test modle freq v2 (Autodesk Fusion 360 design; units mm, degrees)
Autodesk Fusion 360 part; units mm, degrees
ref_plane "WorkPlane1" through (0, 28.011, 0) normal (0, 1, 0) x (0, 0, 1)
sketch "Sketch2" plane through (0, 28.011, 0) normal (0, 1, 0) x (1, 0, 0)
  line L0 (-47.6227, 0.6459) -> (-8.7892, -42.213)
  line L1 (-8.7892, -39.7251) -> (-48.648, 4.2654)
  line L2 (-8.7892, -42.213) -> (0, -42.213)
  line L3 (0, -42.213) -> (0, -36.199)
  line L4 (0, -36.199) -> (-8.7892, -36.199)
  line L5 (-8.7892, -36.199) -> (-8.7892, -42.213)
  line L6 (-47.6227, 0.6459) -> (0, 0.6459)
  line L7 (0, 0.6459) -> (0, 9.3893)
  line L8 (0, 9.3893) -> (-47.6227, 9.3893)
  line L9 (-47.6227, 9.3893) -> (-47.6227, 0.6459)
  constraint parallel L0 L1
  constraint horizontal L2
  constraint vertical L3
  constraint horizontal L4
  constraint vertical L5
  constraint horizontal L6
  constraint vertical L7
  constraint horizontal L8
  constraint vertical L9
  constraint coincident L5 L1.start
extrude "Extrude1" add sketch "Sketch2" along normal blind 3
extrude "Extrude2" add sketch "Sketch2" against normal up to surface (28.011 mm away) contours L1 L6 L9 | L2 L3 L4 L5 | L1 L6 L7 L8 L9
mirror "Mirror1" about plane through (0, 0, 0) normal (1, 0, 0) of bodies 1 merged
mirror "Mirror2" about plane through (0, 0, 0) normal (0, -1, 0) of bodies 1 merged
